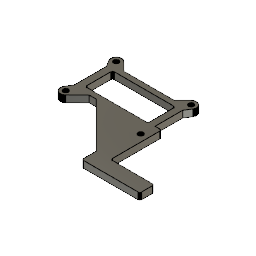
Plate (Autodesk Fusion 360 design; units mm, degrees)
Autodesk Fusion 360 part; units mm, degrees
(part 1 of 3)
sketch "Sketch1" plane through (0, 0, 0) normal (0, 0, 1) x (1, 0, 0)
  line L0 (57.3482, -23.9414) -> (57.363, -23.941)
  line L1 (57.363, -23.941) -> (57.3775, -23.9403)
  line L2 (57.3775, -23.9403) -> (57.3921, -23.9394)
  line L3 (57.3921, -23.9394) -> (57.4066, -23.9383)
  line L4 (57.4066, -23.9383) -> (57.4215, -23.9369)
  line L5 (57.4215, -23.9369) -> (57.436, -23.9352)
  line L6 (57.436, -23.9352) -> (57.4506, -23.9333)
  line L7 (57.4506, -23.9333) -> (57.4649, -23.9311)
  line L8 (57.4649, -23.9311) -> (57.4794, -23.9287)
  line L9 (57.4794, -23.9287) -> (57.494, -23.9261)
  line L10 (57.494, -23.9261) -> (57.5082, -23.9231)
  line L11 (57.5082, -23.9231) -> (57.5225, -23.9199)
  line L12 (57.5225, -23.9199) -> (57.5368, -23.9165)
  line L13 (57.5368, -23.9165) -> (57.5508, -23.9129)
  line L14 (57.5508, -23.9129) -> (57.5651, -23.9089)
  line L15 (57.5651, -23.9089) -> (57.5792, -23.9048)
  line L16 (57.5792, -23.9048) -> (57.5932, -23.9004)
  line L17 (57.5932, -23.9004) -> (57.6069, -23.8957)
  line L18 (57.6069, -23.8957) -> (57.621, -23.8908)
  line L19 (57.621, -23.8908) -> (57.6347, -23.8857)
  line L20 (57.6347, -23.8857) -> (57.6482, -23.8803)
  line L21 (57.6482, -23.8803) -> (57.6617, -23.8747)
  line L22 (57.6617, -23.8747) -> (57.6752, -23.8689)
  line L23 (57.6752, -23.8689) -> (57.6887, -23.8628)
  line L24 (57.6887, -23.8628) -> (57.7019, -23.8565)
  line L25 (57.7019, -23.8565) -> (57.7149, -23.8499)
  line L26 (57.7149, -23.8499) -> (57.7279, -23.8431)
  line L27 (57.7279, -23.8431) -> (57.7408, -23.8362)
  line L28 (57.7408, -23.8362) -> (57.7535, -23.8289)
  line L29 (57.7535, -23.8289) -> (57.7662, -23.8215)
  line L30 (57.7662, -23.8215) -> (57.7787, -23.8138)
  line L31 (57.7787, -23.8138) -> (57.7911, -23.806)
  line L32 (57.7911, -23.806) -> (57.8033, -23.7979)
  line L33 (57.8033, -23.7979) -> (57.8154, -23.7896)
  line L34 (57.8154, -23.7896) -> (57.8273, -23.781)
  line L35 (57.8273, -23.781) -> (57.839, -23.7723)
  line L36 (57.839, -23.7723) -> (57.8506, -23.7634)
  line L37 (57.8506, -23.7634) -> (57.8623, -23.7543)
  line L38 (57.8623, -23.7543) -> (57.8736, -23.745)
  line L39 (57.8736, -23.745) -> (57.8847, -23.7354)
  line L40 (57.8847, -23.7354) -> (57.8956, -23.7257)
  line L41 (57.8956, -23.7257) -> (57.9064, -23.7158)
  line L42 (57.9064, -23.7158) -> (57.917, -23.7057)
  line L43 (57.917, -23.7057) -> (57.9276, -23.6954)
  line L44 (57.9276, -23.6954) -> (57.9379, -23.685)
  line L45 (57.9379, -23.685) -> (57.948, -23.6743)
  line L46 (57.948, -23.6743) -> (57.9578, -23.6635)
  line L47 (57.9578, -23.6635) -> (57.9676, -23.6526)
  line L48 (57.9676, -23.6526) -> (57.9771, -23.6414)
  line L49 (57.9771, -23.6414) -> (57.9863, -23.6301)
  line L50 (57.9863, -23.6301) -> (57.9956, -23.6186)
  line L51 (57.9956, -23.6186) -> (58.0043, -23.607)
  line L52 (58.0043, -23.607) -> (58.0131, -23.5952)
  line L53 (58.0131, -23.5952) -> (58.0218, -23.5833)
  line L54 (58.0218, -23.5833) -> (58.03, -23.5712)
  line L55 (58.03, -23.5712) -> (58.0382, -23.559)
  line L56 (58.0382, -23.559) -> (58.0459, -23.5466)
  line L57 (58.0459, -23.5466) -> (58.0536, -23.5341)
  line L58 (58.0536, -23.5341) -> (58.061, -23.5215)
  line L59 (58.061, -23.5215) -> (58.0684, -23.5087)
  line L60 (58.0684, -23.5087) -> (58.0752, -23.4958)
  line L61 (58.0752, -23.4958) -> (58.0821, -23.4828)
  line L62 (58.0821, -23.4828) -> (58.0885, -23.4697)
  line L63 (58.0885, -23.4697) -> (58.0948, -23.4564)
  line L64 (58.0948, -23.4564) -> (58.1009, -23.4431)
  line L65 (58.1009, -23.4431) -> (58.1067, -23.4297)
  line L66 (58.1067, -23.4297) -> (58.1126, -23.4161)
  line L67 (58.1126, -23.4161) -> (58.1178, -23.4025)
  line L68 (58.1178, -23.4025) -> (58.1229, -23.3887)
  line L69 (58.1229, -23.3887) -> (58.1279, -23.3749)
  line L70 (58.1279, -23.3749) -> (58.1324, -23.361)
  line L71 (58.1324, -23.361) -> (58.1369, -23.347)
  line L72 (58.1369, -23.347) -> (58.1411, -23.333)
  line L73 (58.1411, -23.333) -> (58.1451, -23.3188)
  line L74 (58.1451, -23.3188) -> (58.1485, -23.3047)
  line L75 (58.1485, -23.3047) -> (58.152, -23.2904)
  line L76 (58.152, -23.2904) -> (58.1552, -23.2761)
  line L77 (58.1552, -23.2761) -> (58.1581, -23.2617)
  line L78 (58.1581, -23.2617) -> (58.1607, -23.2473)
  line L79 (58.1607, -23.2473) -> (58.1634, -23.2328)
  line L80 (58.1634, -23.2328) -> (58.1655, -23.2184)
  line L81 (58.1655, -23.2184) -> (58.1673, -23.2038)
  line L82 (58.1673, -23.2038) -> (58.1689, -23.1892)
  line L83 (58.1689, -23.1892) -> (58.1705, -23.1746)
  line L84 (58.1705, -23.1746) -> (58.1716, -23.16)
  line L85 (58.1716, -23.16) -> (58.1723, -23.1454)
  line L86 (58.1723, -23.1454) -> (58.1731, -23.1307)
  line L87 (58.1731, -23.1307) -> (58.1734, -23.1161)
  line L88 (58.1734, -23.1161) -> (58.1737, -23.1014)
  line L89 (58.1737, -23.1014) -> (58.1737, -18.0611)
  line L90 (58.1737, -18.0611) -> (58.1734, -18.0465)
  line L91 (58.1734, -18.0465) -> (58.1731, -18.0318)
  line L92 (58.1731, -18.0318) -> (58.1723, -18.0171)
  line L93 (58.1723, -18.0171) -> (58.1716, -18.0025)
  line L94 (58.1716, -18.0025) -> (58.1705, -17.9879)
  line L95 (58.1705, -17.9879) -> (58.1689, -17.9733)
  line L96 (58.1689, -17.9733) -> (58.1673, -17.9588)
  line L97 (58.1673, -17.9588) -> (58.1655, -17.9442)
  line L98 (58.1655, -17.9442) -> (58.1634, -17.9297)
  line L99 (58.1634, -17.9297) -> (58.1607, -17.9153)
  line L100 (58.1607, -17.9153) -> (58.1581, -17.9008)
  line L101 (58.1581, -17.9008) -> (58.1552, -17.8865)
  line L102 (58.1552, -17.8865) -> (58.152, -17.8722)
  line L103 (58.152, -17.8722) -> (58.1485, -17.8579)
  line L104 (58.1485, -17.8579) -> (58.1451, -17.8437)
  line L105 (58.1451, -17.8437) -> (58.1411, -17.8296)
  line L106 (58.1411, -17.8296) -> (58.1369, -17.8155)
  line L107 (58.1369, -17.8155) -> (58.1324, -17.8015)
  line L108 (58.1324, -17.8015) -> (58.1279, -17.7876)
  line L109 (58.1279, -17.7876) -> (58.1229, -17.7738)
  line L110 (58.1229, -17.7738) -> (58.1178, -17.7601)
  line L111 (58.1178, -17.7601) -> (58.1126, -17.7464)
  line L112 (58.1126, -17.7464) -> (58.1067, -17.7329)
  line L113 (58.1067, -17.7329) -> (58.1009, -17.7194)
  line L114 (58.1009, -17.7194) -> (58.0948, -17.7061)
  line L115 (58.0948, -17.7061) -> (58.0885, -17.6929)
  line L116 (58.0885, -17.6929) -> (58.0821, -17.6797)
  line L117 (58.0821, -17.6797) -> (58.0752, -17.6667)
  line L118 (58.0752, -17.6667) -> (58.0684, -17.6538)
  line L119 (58.0684, -17.6538) -> (58.061, -17.6411)
  line L120 (58.061, -17.6411) -> (58.0536, -17.6285)
  line L121 (58.0536, -17.6285) -> (58.0459, -17.616)
  line L122 (58.0459, -17.616) -> (58.0382, -17.6036)
  line L123 (58.0382, -17.6036) -> (58.03, -17.5914)
  line L124 (58.03, -17.5914) -> (58.0218, -17.5793)
  line L125 (58.0218, -17.5793) -> (58.0131, -17.5674)
  line L126 (58.0131, -17.5674) -> (58.0043, -17.5556)
  line L127 (58.0043, -17.5556) -> (57.9956, -17.5439)
  line L128 (57.9956, -17.5439) -> (57.9863, -17.5325)
  line L129 (57.9863, -17.5325) -> (57.9771, -17.5211)
  line L130 (57.9771, -17.5211) -> (57.9676, -17.51)
  line L131 (57.9676, -17.51) -> (57.9578, -17.499)
  line L132 (57.9578, -17.499) -> (57.948, -17.4882)
  line L133 (57.948, -17.4882) -> (57.9379, -17.4776)
  line L134 (57.9379, -17.4776) -> (57.9276, -17.4671)
  line L135 (57.9276, -17.4671) -> (57.917, -17.4568)
  line L136 (57.917, -17.4568) -> (57.9064, -17.4467)
  line L137 (57.9064, -17.4467) -> (57.8956, -17.4368)
  line L138 (57.8956, -17.4368) -> (57.8847, -17.4271)
  line L139 (57.8847, -17.4271) -> (57.8736, -17.4176)
  line L140 (57.8736, -17.4176) -> (57.8623, -17.4083)
  line L141 (57.8623, -17.4083) -> (57.8506, -17.3992)
  line L142 (57.8506, -17.3992) -> (57.839, -17.3902)
  line L143 (57.839, -17.3902) -> (57.8273, -17.3815)
  line L144 (57.8273, -17.3815) -> (57.8154, -17.373)
  line L145 (57.8154, -17.373) -> (57.8033, -17.3647)
  line L146 (57.8033, -17.3647) -> (57.7911, -17.3566)
  line L147 (57.7911, -17.3566) -> (57.7787, -17.3487)
  line L148 (57.7787, -17.3487) -> (57.7662, -17.3411)
  line L149 (57.7662, -17.3411) -> (57.7535, -17.3336)
  line L150 (57.7535, -17.3336) -> (57.7408, -17.3264)
  line L151 (57.7408, -17.3264) -> (57.7279, -17.3194)
  line L152 (57.7279, -17.3194) -> (57.7149, -17.3126)
  line L153 (57.7149, -17.3126) -> (57.7019, -17.3061)
  line L154 (57.7019, -17.3061) -> (57.6887, -17.2998)
  line L155 (57.6887, -17.2998) -> (57.6752, -17.2937)
  line L156 (57.6752, -17.2937) -> (57.6617, -17.2878)
  line L157 (57.6617, -17.2878) -> (57.6482, -17.2822)
  line L158 (57.6482, -17.2822) -> (57.6347, -17.2769)
  line L159 (57.6347, -17.2769) -> (57.621, -17.2717)
  line L160 (57.621, -17.2717) -> (57.6069, -17.2668)
  line L161 (57.6069, -17.2668) -> (57.5932, -17.2622)
  line L162 (57.5932, -17.2622) -> (57.5792, -17.2578)
  line L163 (57.5792, -17.2578) -> (57.5651, -17.2536)
  line L164 (57.5651, -17.2536) -> (57.5508, -17.2497)
  line L165 (57.5508, -17.2497) -> (57.5368, -17.246)
  line L166 (57.5368, -17.246) -> (57.5225, -17.2426)
  line L167 (57.5225, -17.2426) -> (57.5082, -17.2394)
  line L168 (57.5082, -17.2394) -> (57.494, -17.2365)
  line L169 (57.494, -17.2365) -> (57.4794, -17.2338)
  line L170 (57.4794, -17.2338) -> (57.4649, -17.2314)
  line L171 (57.4649, -17.2314) -> (57.4506, -17.2292)
  line L172 (57.4506, -17.2292) -> (57.436, -17.2273)
  line L173 (57.436, -17.2273) -> (57.4215, -17.2257)
  line L174 (57.4215, -17.2257) -> (57.4066, -17.2243)
  line L175 (57.4066, -17.2243) -> (57.3921, -17.2231)
  line L176 (57.3921, -17.2231) -> (57.3775, -17.2222)
  line L177 (57.3775, -17.2222) -> (57.363, -17.2216)
  line L178 (57.363, -17.2216) -> (57.3482, -17.2212)
  line L179 (57.3482, -17.2212) -> (57.3336, -17.2211)
  line L180 (57.3336, -17.2211) -> (38.8562, -17.2211)
  line L181 (38.8562, -17.2211) -> (38.8379, -17.2209)
  line L182 (38.8379, -17.2209) -> (38.8231, -17.2205)
  line L183 (38.8231, -17.2205) -> (38.8083, -17.2199)
  line L184 (38.8083, -17.2199) -> (38.7937, -17.219)
  line L185 (38.7937, -17.219) -> (38.7792, -17.2178)
  line L186 (38.7792, -17.2178) -> (38.7646, -17.2164)
  line L187 (38.7646, -17.2164) -> (38.7501, -17.2148)
  line L188 (38.7501, -17.2148) -> (38.7355, -17.2129)
  line L189 (38.7355, -17.2129) -> (38.721, -17.2107)
  line L190 (38.721, -17.2107) -> (38.7064, -17.2082)
  line L191 (38.7064, -17.2082) -> (38.6921, -17.2056)
  line L192 (38.6921, -17.2056) -> (38.6779, -17.2027)
  line L193 (38.6779, -17.2027) -> (38.6636, -17.1995)
  line L194 (38.6636, -17.1995) -> (38.649, -17.196)
  line L195 (38.649, -17.196) -> (38.635, -17.1924)
  line L196 (38.635, -17.1924) -> (38.621, -17.1885)
  line L197 (38.621, -17.1885) -> (38.6067, -17.1843)
  line L198 (38.6067, -17.1843) -> (38.5929, -17.18)
  line L199 (38.5929, -17.18) -> (38.5789, -17.1753)
  line L200 (38.5789, -17.1753) -> (38.5651, -17.1704)
  line L201 (38.5651, -17.1704) -> (38.5514, -17.1652)
  line L202 (38.5514, -17.1652) -> (38.5379, -17.1599)
  line L203 (38.5379, -17.1599) -> (38.5241, -17.1542)
  line L204 (38.5241, -17.1542) -> (38.5109, -17.1484)
  line L205 (38.5109, -17.1484) -> (38.4974, -17.1423)
  line L206 (38.4974, -17.1423) -> (38.4842, -17.136)
  line L207 (38.4842, -17.136) -> (38.4709, -17.1294)
  line L208 (38.4709, -17.1294) -> (38.4582, -17.1228)
  line L209 (38.4582, -17.1228) -> (38.445, -17.1157)
  line L210 (38.445, -17.1157) -> (38.4326, -17.1085)
  line L211 (38.4326, -17.1085) -> (38.4199, -17.1011)
  line L212 (38.4199, -17.1011) -> (38.4072, -17.0934)
  line L213 (38.4072, -17.0934) -> (38.395, -17.0855)
  line L214 (38.395, -17.0855) -> (38.3826, -17.0774)
  line L215 (38.3826, -17.0774) -> (38.3707, -17.0692)
  line L216 (38.3707, -17.0692) -> (38.3585, -17.0606)
  line L217 (38.3585, -17.0606) -> (38.3469, -17.0519)
  line L218 (38.3469, -17.0519) -> (38.3352, -17.0429)
  line L219 (38.3352, -17.0429) -> (38.3238, -17.0338)
  line L220 (38.3238, -17.0338) -> (38.3125, -17.0246)
  line L221 (38.3125, -17.0246) -> (38.3013, -17.0149)
  line L222 (38.3013, -17.0149) -> (38.2902, -17.0053)
  line L223 (38.2902, -17.0053) -> (38.2794, -16.9953)
  line L224 (38.2794, -16.9953) -> (38.2688, -16.9853)
  line L225 (38.2688, -16.9853) -> (38.2585, -16.975)
  line L226 (38.2585, -16.975) -> (38.2482, -16.9645)
  line L227 (38.2482, -16.9645) -> (38.2381, -16.954)
  line L228 (38.2381, -16.954) -> (38.2281, -16.943)
  line L229 (38.2281, -16.943) -> (38.2185, -16.9322)
  line L230 (38.2185, -16.9322) -> (38.2087, -16.9208)
  line L231 (38.2087, -16.9208) -> (38.1995, -16.9097)
  line L232 (38.1995, -16.9097) -> (38.1905, -16.8982)
  line L233 (38.1905, -16.8982) -> (38.1815, -16.8865)
  line L234 (38.1815, -16.8865) -> (38.1728, -16.8748)
  line L235 (38.1728, -16.8748) -> (38.1643, -16.8628)
  line L236 (38.1643, -16.8628) -> (38.1561, -16.8508)
  line L237 (38.1561, -16.8508) -> (38.1479, -16.8385)
  line L238 (38.1479, -16.8385) -> (38.14, -16.8262)
  line L239 (38.14, -16.8262) -> (38.1323, -16.8137)
  line L240 (38.1323, -16.8137) -> (38.1249, -16.801)
  line L241 (38.1249, -16.801) -> (38.1177, -16.7884)
  line L242 (38.1177, -16.7884) -> (38.1106, -16.7752)
  line L243 (38.1106, -16.7752) -> (38.104, -16.7625)
  line L244 (38.104, -16.7625) -> (38.0974, -16.7493)
  line L245 (38.0974, -16.7493) -> (38.091, -16.7361)
  line L246 (38.091, -16.7361) -> (38.0849, -16.7226)
  line L247 (38.0849, -16.7226) -> (38.0791, -16.7093)
  line L248 (38.0791, -16.7093) -> (38.0735, -16.6956)
  line L249 (38.0735, -16.6956) -> (38.0683, -16.6821)
  line L250 (38.0683, -16.6821) -> (38.063, -16.6683)
  line L251 (38.063, -16.6683) -> (38.0582, -16.6545)
  line L252 (38.0582, -16.6545) -> (38.0534, -16.6405)
  line L253 (38.0534, -16.6405) -> (38.0492, -16.6266)
  line L254 (38.0492, -16.6266) -> (38.045, -16.6125)
  line L255 (38.045, -16.6125) -> (38.041, -16.5984)
  line L256 (38.041, -16.5984) -> (38.0373, -16.5844)
  line L257 (38.0373, -16.5844) -> (38.0339, -16.5699)
  line L258 (38.0339, -16.5699) -> (38.0307, -16.5555)
  line L259 (38.0307, -16.5555) -> (38.0278, -16.5414)
  line L260 (38.0278, -16.5414) -> (38.0251, -16.527)
  line L261 (38.0251, -16.527) -> (38.0227, -16.5123)
  line L262 (38.0227, -16.5123) -> (38.0206, -16.4979)
  line L263 (38.0206, -16.4979) -> (38.0188, -16.4834)
  line L264 (38.0188, -16.4834) -> (38.0169, -16.4687)
  line L265 (38.0169, -16.4687) -> (38.0156, -16.4543)
  line L266 (38.0156, -16.4543) -> (38.0145, -16.4396)
  line L267 (38.0145, -16.4396) -> (38.0135, -16.4252)
  line L268 (38.0135, -16.4252) -> (38.013, -16.4103)
  line L269 (38.013, -16.4103) -> (38.0124, -16.3956)
  line L270 (38.0124, -16.3956) -> (38.0124, -16.3773)
  line L271 (38.0124, -16.3773) -> (38.0124, 5.4603)
  line L272 (38.0124, 5.4603) -> (38.0122, 5.475)
  line L273 (38.0122, 5.475) -> (38.0119, 5.4897)
  line L274 (38.0119, 5.4897) -> (38.0111, 5.5043)
  line L275 (38.0111, 5.5043) -> (38.0103, 5.5189)
  line L276 (38.0103, 5.5189) -> (38.0092, 5.5335)
  line L277 (38.0092, 5.5335) -> (38.0077, 5.5482)
  line L278 (38.0077, 5.5482) -> (38.0061, 5.5627)
  line L279 (38.0061, 5.5627) -> (38.0042, 5.5773)
  line L280 (38.0042, 5.5773) -> (38.0021, 5.5918)
  line L281 (38.0021, 5.5918) -> (37.9995, 5.6062)
  line L282 (37.9995, 5.6062) -> (37.9968, 5.6206)
  line L283 (37.9968, 5.6206) -> (37.9939, 5.635)
  line L284 (37.9939, 5.635) -> (37.9907, 5.6493)
  line L285 (37.9907, 5.6493) -> (37.9873, 5.6636)
  line L286 (37.9873, 5.6636) -> (37.9838, 5.6777)
  line L287 (37.9838, 5.6777) -> (37.9799, 5.6919)
  line L288 (37.9799, 5.6919) -> (37.9756, 5.706)
  line L289 (37.9756, 5.706) -> (37.9711, 5.7199)
  line L290 (37.9711, 5.7199) -> (37.9667, 5.7338)
  line L291 (37.9667, 5.7338) -> (37.9616, 5.7476)
  line L292 (37.9616, 5.7476) -> (37.9566, 5.7614)
  line L293 (37.9566, 5.7614) -> (37.9513, 5.775)
  line L294 (37.9513, 5.775) -> (37.9455, 5.7886)
  line L295 (37.9455, 5.7886) -> (37.9397, 5.802)
  line L296 (37.9397, 5.802) -> (37.9336, 5.8154)
  line L297 (37.9336, 5.8154) -> (37.9272, 5.8286)
  line L298 (37.9272, 5.8286) -> (37.9209, 5.8417)
  line L299 (37.9209, 5.8417) -> (37.914, 5.8547)
  line L300 (37.914, 5.8547) -> (37.9071, 5.8676)
  line L301 (37.9071, 5.8676) -> (37.8997, 5.8804)
  line L302 (37.8997, 5.8804) -> (37.8923, 5.893)
  line L303 (37.8923, 5.893) -> (37.8846, 5.9055)
  line L304 (37.8846, 5.9055) -> (37.877, 5.9179)
  line L305 (37.877, 5.9179) -> (37.8688, 5.9301)
  line L306 (37.8688, 5.9301) -> (37.8606, 5.9422)
  line L307 (37.8606, 5.9422) -> (37.8518, 5.9541)
  line L308 (37.8518, 5.9541) -> (37.8431, 5.9659)
  line L309 (37.8431, 5.9659) -> (37.8344, 5.9775)
  line L310 (37.8344, 5.9775) -> (37.8251, 5.989)
  line L311 (37.8251, 5.989) -> (37.8158, 6.0003)
  line L312 (37.8158, 6.0003) -> (37.8063, 6.0115)
  line L313 (37.8063, 6.0115) -> (37.7965, 6.0224)
  line L314 (37.7965, 6.0224) -> (37.7867, 6.0332)
  line L315 (37.7867, 6.0332) -> (37.7767, 6.0439)
  line L316 (37.7767, 6.0439) -> (37.7664, 6.0544)
  line L317 (37.7664, 6.0544) -> (37.7558, 6.0646)
  line L318 (37.7558, 6.0646) -> (37.7452, 6.0747)
  line L319 (37.7452, 6.0747) -> (37.7343, 6.0846)
  line L320 (37.7343, 6.0846) -> (37.7235, 6.0943)
  line L321 (37.7235, 6.0943) -> (37.7124, 6.1039)
  line L322 (37.7124, 6.1039) -> (37.701, 6.1132)
  line L323 (37.701, 6.1132) -> (37.6894, 6.1223)
  line L324 (37.6894, 6.1223) -> (37.6777, 6.1312)
  line L325 (37.6777, 6.1312) -> (37.6661, 6.1399)
  line L326 (37.6661, 6.1399) -> (37.6542, 6.1485)
  line L327 (37.6542, 6.1485) -> (37.642, 6.1568)
  line L328 (37.642, 6.1568) -> (37.6298, 6.1649)
  line L329 (37.6298, 6.1649) -> (37.6174, 6.1727)
  line L330 (37.6174, 6.1727) -> (37.605, 6.1804)
  line L331 (37.605, 6.1804) -> (37.5923, 6.1878)
  line L332 (37.5923, 6.1878) -> (37.5796, 6.1951)
  line L333 (37.5796, 6.1951) -> (37.5666, 6.202)
  line L334 (37.5666, 6.202) -> (37.5536, 6.2088)
  line L335 (37.5536, 6.2088) -> (37.5407, 6.2154)
  line L336 (37.5407, 6.2154) -> (37.5274, 6.2217)
  line L337 (37.5274, 6.2217) -> (37.5139, 6.2278)
  line L338 (37.5139, 6.2278) -> (37.5005, 6.2336)
  line L339 (37.5005, 6.2336) -> (37.487, 6.2392)
  line L340 (37.487, 6.2392) -> (37.4735, 6.2446)
  line L341 (37.4735, 6.2446) -> (37.4597, 6.2497)
  line L342 (37.4597, 6.2497) -> (37.4457, 6.2546)
  line L343 (37.4457, 6.2546) -> (37.4319, 6.2593)
  line L344 (37.4319, 6.2593) -> (37.4179, 6.2637)
  line L345 (37.4179, 6.2637) -> (37.4039, 6.2678)
  line L346 (37.4039, 6.2678) -> (37.3896, 6.2718)
  line L347 (37.3896, 6.2718) -> (37.3756, 6.2754)
  line L348 (37.3756, 6.2754) -> (37.3613, 6.2789)
  line L349 (37.3613, 6.2789) -> (37.347, 6.282)
  line L350 (37.347, 6.282) -> (37.3327, 6.285)
  line L351 (37.3327, 6.285) -> (37.3182, 6.2876)
  line L352 (37.3182, 6.2876) -> (37.3036, 6.29)
  line L353 (37.3036, 6.29) -> (37.2893, 6.2922)
  line L354 (37.2893, 6.2922) -> (37.2748, 6.2941)
  line L355 (37.2748, 6.2941) -> (37.2602, 6.2958)
  line L356 (37.2602, 6.2958) -> (37.2454, 6.2972)
  line L357 (37.2454, 6.2972) -> (37.2308, 6.2983)
  line L358 (37.2308, 6.2983) -> (37.2163, 6.2992)
  line L359 (37.2163, 6.2992) -> (37.2017, 6.2999)
  line L360 (37.2017, 6.2999) -> (37.1869, 6.3003)
  line L361 (37.1869, 6.3003) -> (37.1724, 6.3004)
  line L362 (37.1724, 6.3004) -> (34.9671, 6.3004)
  line L363 (34.9671, 6.3004) -> (34.9671, 19.1018)
  line L364 (34.9671, 19.1018) -> (36.7893, 21.976)
  line L365 (36.7893, 21.976) -> (36.8123, 22.0135)
  line L366 (36.8123, 22.0135) -> (36.8348, 22.0514)
  line L367 (36.8348, 22.0514) -> (36.8562, 22.0896)
  line L368 (36.8562, 22.0896) -> (36.8774, 22.1283)
  line L369 (36.8774, 22.1283) -> (36.8977, 22.1673)
  line L370 (36.8977, 22.1673) -> (36.9173, 22.2067)
  line L371 (36.9173, 22.2067) -> (36.9361, 22.2464)
  line L372 (36.9361, 22.2464) -> (36.9544, 22.2864)
  line L373 (36.9544, 22.2864) -> (36.9721, 22.3267)
  line L374 (36.9721, 22.3267) -> (36.9888, 22.3674)
  line L375 (36.9888, 22.3674) -> (37.0049, 22.4083)
  line L376 (37.0049, 22.4083) -> (37.0202, 22.4495)
  line L377 (37.0202, 22.4495) -> (37.0351, 22.491)
  line L378 (37.0351, 22.491) -> (37.0491, 22.5327)
  line L379 (37.0491, 22.5327) -> (37.0623, 22.5746)
  line L380 (37.0623, 22.5746) -> (37.0747, 22.6168)
  line L381 (37.0747, 22.6168) -> (37.0864, 22.6592)
  line L382 (37.0864, 22.6592) -> (37.0975, 22.7018)
  line L383 (37.0975, 22.7018) -> (37.1078, 22.7445)
  line L384 (37.1078, 22.7445) -> (37.1173, 22.7875)
  line L385 (37.1173, 22.7875) -> (37.1261, 22.8306)
  line L386 (37.1261, 22.8306) -> (37.134, 22.8738)
  line L387 (37.134, 22.8738) -> (37.1412, 22.9172)
  line L388 (37.1412, 22.9172) -> (37.1478, 22.9607)
  line L389 (37.1478, 22.9607) -> (37.1536, 23.0043)
  line L390 (37.1536, 23.0043) -> (37.1586, 23.048)
  line L391 (37.1586, 23.048) -> (37.1628, 23.0918)
  line L392 (37.1628, 23.0918) -> (37.1663, 23.1356)
  line L393 (37.1663, 23.1356) -> (37.1689, 23.1795)
  line L394 (37.1689, 23.1795) -> (37.1708, 23.2235)
  line L395 (37.1708, 23.2235) -> (37.1718, 23.2675)
  line L396 (37.1718, 23.2675) -> (37.1724, 23.3114)
  line L397 (37.1724, 23.3114) -> (37.1718, 23.3554)
  line L398 (37.1718, 23.3554) -> (37.1708, 23.3994)
  line L399 (37.1708, 23.3994) -> (37.1689, 23.4433)
  line L400 (37.1689, 23.4433) -> (37.1663, 23.4872)
  line L401 (37.1663, 23.4872) -> (37.1628, 23.5311)
  line L402 (37.1628, 23.5311) -> (37.1586, 23.5749)
  line L403 (37.1586, 23.5749) -> (37.1536, 23.6186)
  line L404 (37.1536, 23.6186) -> (37.1478, 23.6622)
  line L405 (37.1478, 23.6622) -> (37.1412, 23.7057)
  line L406 (37.1412, 23.7057) -> (37.134, 23.7491)
  line L407 (37.134, 23.7491) -> (37.1261, 23.7923)
  line L408 (37.1261, 23.7923) -> (37.1173, 23.8354)
  line L409 (37.1173, 23.8354) -> (37.1078, 23.8784)
  line L410 (37.1078, 23.8784) -> (37.0975, 23.9211)
  line L411 (37.0975, 23.9211) -> (37.0864, 23.9637)
  line L412 (37.0864, 23.9637) -> (37.0747, 24.0061)
  line L413 (37.0747, 24.0061) -> (37.0623, 24.0483)
  line L414 (37.0623, 24.0483) -> (37.0491, 24.0902)
  line L415 (37.0491, 24.0902) -> (37.0351, 24.1319)
  line L416 (37.0351, 24.1319) -> (37.0202, 24.1734)
  line L417 (37.0202, 24.1734) -> (37.0049, 24.2146)
  line L418 (37.0049, 24.2146) -> (36.9888, 24.2555)
  line L419 (36.9888, 24.2555) -> (36.9721, 24.2962)
  line L420 (36.9721, 24.2962) -> (36.9544, 24.3365)
  line L421 (36.9544, 24.3365) -> (36.9361, 24.3765)
  line L422 (36.9361, 24.3765) -> (36.9173, 24.4162)
  line L423 (36.9173, 24.4162) -> (36.8977, 24.4556)
  line L424 (36.8977, 24.4556) -> (36.8774, 24.4946)
  line L425 (36.8774, 24.4946) -> (36.8562, 24.5333)
  line L426 (36.8562, 24.5333) -> (36.8348, 24.5715)
  line L427 (36.8348, 24.5715) -> (36.8123, 24.6094)
  line L428 (36.8123, 24.6094) -> (36.7893, 24.6469)
  line L429 (36.7893, 24.6469) -> (36.7657, 24.684)
  line L430 (36.7657, 24.684) -> (36.7414, 24.7207)
  line L431 (36.7414, 24.7207) -> (36.7165, 24.757)
  line L432 (36.7165, 24.757) -> (36.6911, 24.7928)
  line L433 (36.6911, 24.7928) -> (36.6649, 24.8281)
  line L434 (36.6649, 24.8281) -> (36.6382, 24.863)
  line L435 (36.6382, 24.863) -> (36.6107, 24.8974)
  line L436 (36.6107, 24.8974) -> (36.5826, 24.9314)
  line L437 (36.5826, 24.9314) -> (36.554, 24.9648)
  line L438 (36.554, 24.9648) -> (36.5249, 24.9978)
  line L439 (36.5249, 24.9978) -> (36.4953, 25.0302)
  line L440 (36.4953, 25.0302) -> (36.4649, 25.0621)
  line L441 (36.4649, 25.0621) -> (36.4342, 25.0935)
  line L442 (36.4342, 25.0935) -> (36.4027, 25.1243)
  line L443 (36.4027, 25.1243) -> (36.3709, 25.1546)
  line L444 (36.3709, 25.1546) -> (36.3384, 25.1843)
  line L445 (36.3384, 25.1843) -> (36.3056, 25.2134)
  line L446 (36.3056, 25.2134) -> (36.272, 25.242)
  line L447 (36.272, 25.242) -> (36.2381, 25.27)
  line L448 (36.2381, 25.27) -> (36.2037, 25.2973)
  line L449 (36.2037, 25.2973) -> (36.1688, 25.3241)
  line L450 (36.1688, 25.3241) -> (36.1334, 25.3503)
  line L451 (36.1334, 25.3503) -> (36.0976, 25.3758)
  line L452 (36.0976, 25.3758) -> (36.0614, 25.4007)
  line L453 (36.0614, 25.4007) -> (36.0246, 25.425)
  line L454 (36.0246, 25.425) -> (35.9876, 25.4487)
  line L455 (35.9876, 25.4487) -> (35.95, 25.4716)
  line L456 (35.95, 25.4716) -> (35.9122, 25.494)
  line L457 (35.9122, 25.494) -> (35.8741, 25.5156)
  line L458 (35.8741, 25.5156) -> (35.8352, 25.5366)
  line L459 (35.8352, 25.5366) -> (35.7963, 25.5569)
  line L460 (35.7963, 25.5569) -> (35.7568, 25.5766)
  line L461 (35.7568, 25.5766) -> (35.7172, 25.5955)
  line L462 (35.7172, 25.5955) -> (35.6772, 25.6137)
  line L463 (35.6772, 25.6137) -> (35.6367, 25.6313)
  line L464 (35.6367, 25.6313) -> (35.5962, 25.6481)
  line L465 (35.5962, 25.6481) -> (35.5552, 25.6642)
  line L466 (35.5552, 25.6642) -> (35.514, 25.6796)
  line L467 (35.514, 25.6796) -> (35.4727, 25.6943)
  line L468 (35.4727, 25.6943) -> (35.4309, 25.7083)
  line L469 (35.4309, 25.7083) -> (35.3891, 25.7215)
  line L470 (35.3891, 25.7215) -> (35.3467, 25.734)
  line L471 (35.3467, 25.734) -> (35.3044, 25.7457)
  line L472 (35.3044, 25.7457) -> (35.2618, 25.7567)
  line L473 (35.2618, 25.7567) -> (35.219, 25.767)
  line L474 (35.219, 25.767) -> (35.1761, 25.7765)
  line L475 (35.1761, 25.7765) -> (35.133, 25.7853)
  line L476 (35.133, 25.7853) -> (35.0898, 25.7933)
  line L477 (35.0898, 25.7933) -> (35.0464, 25.8006)
  line L478 (35.0464, 25.8006) -> (35.0028, 25.8071)
  line L479 (35.0028, 25.8071) -> (34.9594, 25.8128)
  line L480 (34.9594, 25.8128) -> (34.9155, 25.8178)
  line L481 (34.9155, 25.8178) -> (34.8718, 25.822)
  line L482 (34.8718, 25.822) -> (34.8279, 25.8255)
  line L483 (34.8279, 25.8255) -> (34.784, 25.8281)
  line L484 (34.784, 25.8281) -> (34.7401, 25.8301)
  line L485 (34.7401, 25.8301) -> (34.6961, 25.8312)
  line L486 (34.6961, 25.8312) -> (34.6522, 25.8316)
  line L487 (34.6522, 25.8316) -> (34.6083, 25.8312)
  line L488 (34.6083, 25.8312) -> (34.5641, 25.8301)
  line L489 (34.5641, 25.8301) -> (34.5202, 25.8281)
  line L490 (34.5202, 25.8281) -> (34.4763, 25.8255)
  line L491 (34.4763, 25.8255) -> (34.4326, 25.822)
  line L492 (34.4326, 25.822) -> (34.3887, 25.8178)
  line L493 (34.3887, 25.8178) -> (34.345, 25.8128)
  line L494 (34.345, 25.8128) -> (34.3014, 25.8071)
  line L495 (34.3014, 25.8071) -> (34.258, 25.8006)
  line L496 (34.258, 25.8006) -> (34.2146, 25.7933)
  line L497 (34.2146, 25.7933) -> (34.1712, 25.7853)
  line L498 (34.1712, 25.7853) -> (34.1281, 25.7765)
  line L499 (34.1281, 25.7765) -> (34.0852, 25.767)
  line L500 (34.0852, 25.767) -> (34.0424, 25.7567)
  line L501 (34.0424, 25.7567) -> (33.9998, 25.7457)
  line L502 (33.9998, 25.7457) -> (33.9574, 25.734)
  line L503 (33.9574, 25.734) -> (33.9154, 25.7215)
  line L504 (33.9154, 25.7215) -> (33.8733, 25.7083)
  line L505 (33.8733, 25.7083) -> (33.8317, 25.6943)
  line L506 (33.8317, 25.6943) -> (33.7902, 25.6796)
  line L507 (33.7902, 25.6796) -> (33.7489, 25.6642)
  line L508 (33.7489, 25.6642) -> (33.7082, 25.6481)
  line L509 (33.7082, 25.6481) -> (33.6674, 25.6313)
  line L510 (33.6674, 25.6313) -> (33.6272, 25.6137)
  line L511 (33.6272, 25.6137) -> (33.587, 25.5955)
  line L512 (33.587, 25.5955) -> (33.5473, 25.5766)
  line L513 (33.5473, 25.5766) -> (33.5079, 25.5569)
  line L514 (33.5079, 25.5569) -> (33.469, 25.5366)
  line L515 (33.469, 25.5366) -> (33.4304, 25.5156)
  line L516 (33.4304, 25.5156) -> (33.392, 25.494)
  line L517 (33.392, 25.494) -> (33.3542, 25.4716)
  line L518 (33.3542, 25.4716) -> (33.3166, 25.4487)
  line L519 (33.3166, 25.4487) -> (33.2796, 25.425)
  line L520 (33.2796, 25.425) -> (33.2428, 25.4007)
  line L521 (33.2428, 25.4007) -> (33.2065, 25.3758)
  line L522 (33.2065, 25.3758) -> (33.1708, 25.3503)
  line L523 (33.1708, 25.3503) -> (33.1354, 25.3241)
  line L524 (33.1354, 25.3241) -> (33.1007, 25.2973)
  line L525 (33.1007, 25.2973) -> (33.066, 25.27)
  line L526 (33.066, 25.27) -> (33.0322, 25.242)
  line L527 (33.0322, 25.242) -> (32.9988, 25.2134)
  line L528 (32.9988, 25.2134) -> (32.9658, 25.1843)
  line L529 (32.9658, 25.1843) -> (32.9335, 25.1546)
  line L530 (32.9335, 25.1546) -> (32.9015, 25.1243)
  line L531 (32.9015, 25.1243) -> (28.902, 21.2113)
  line L532 (28.902, 21.2113) -> (5.75, 21.2113)
  line L533 (5.75, 21.2113) -> (1.7506, 25.1243)
  line L534 (1.7506, 25.1243) -> (1.7187, 25.1546)
  line L535 (1.7187, 25.1546) -> (1.6863, 25.1843)
  line L536 (1.6863, 25.1843) -> (1.6534, 25.2134)
  line L537 (1.6534, 25.2134) -> (1.6199, 25.242)
  line L538 (1.6199, 25.242) -> (1.586, 25.27)
  line L539 (1.586, 25.27) -> (1.5516, 25.2973)
  line L540 (1.5516, 25.2973) -> (1.5167, 25.3241)
  line L541 (1.5167, 25.3241) -> (1.4813, 25.3503)
  line L542 (1.4813, 25.3503) -> (1.4455, 25.3758)
  line L543 (1.4455, 25.3758) -> (1.4093, 25.4007)
  line L544 (1.4093, 25.4007) -> (1.3726, 25.425)
  line L545 (1.3726, 25.425) -> (1.3355, 25.4487)
  line L546 (1.3355, 25.4487) -> (1.298, 25.4716)
  line L547 (1.298, 25.4716) -> (1.2601, 25.494)
  line L548 (1.2601, 25.494) -> (1.2218, 25.5156)
  line L549 (1.2218, 25.5156) -> (1.1831, 25.5366)
  line L550 (1.1831, 25.5366) -> (1.1441, 25.5569)
  line L551 (1.1441, 25.5569) -> (1.1048, 25.5766)
  line L552 (1.1048, 25.5766) -> (1.0651, 25.5955)
  line L553 (1.0651, 25.5955) -> (1.025, 25.6137)
  line L554 (1.025, 25.6137) -> (0.9847, 25.6313)
  line L555 (0.9847, 25.6313) -> (0.9441, 25.6481)
  line L556 (0.9441, 25.6481) -> (0.9031, 25.6642)
  line L557 (0.9031, 25.6642) -> (0.8619, 25.6796)
  line L558 (0.8619, 25.6796) -> (0.8205, 25.6943)
  line L559 (0.8205, 25.6943) -> (0.7788, 25.7083)
  line L560 (0.7788, 25.7083) -> (0.7368, 25.7215)
  line L561 (0.7368, 25.7215) -> (0.6946, 25.734)
  line L562 (0.6946, 25.734) -> (0.6523, 25.7457)
  line L563 (0.6523, 25.7457) -> (0.6097, 25.7567)
  line L564 (0.6097, 25.7567) -> (0.5669, 25.767)
  line L565 (0.5669, 25.767) -> (0.524, 25.7765)
  line L566 (0.524, 25.7765) -> (0.4809, 25.7853)
  line L567 (0.4809, 25.7853) -> (0.4376, 25.7933)
  line L568 (0.4376, 25.7933) -> (0.3942, 25.8006)
  line L569 (0.3942, 25.8006) -> (0.3507, 25.8071)
  line L570 (0.3507, 25.8071) -> (0.3071, 25.8128)
  line L571 (0.3071, 25.8128) -> (0.2634, 25.8178)
  line L572 (0.2634, 25.8178) -> (0.2196, 25.822)
  line L573 (0.2196, 25.822) -> (0.1758, 25.8255)
  line L574 (0.1758, 25.8255) -> (0.1319, 25.8281)
  line L575 (0.1319, 25.8281) -> (0.088, 25.8301)
  line L576 (0.088, 25.8301) -> (0.044, 25.8312)
  line L577 (0.044, 25.8312) -> (0, 25.8316)
  line L578 (0, 25.8316) -> (-0.044, 25.8312)
  line L579 (-0.044, 25.8312) -> (-0.088, 25.8301)
  line L580 (-0.088, 25.8301) -> (-0.1319, 25.8281)
  line L581 (-0.1319, 25.8281) -> (-0.1758, 25.8255)
  line L582 (-0.1758, 25.8255) -> (-0.2196, 25.822)
  line L583 (-0.2196, 25.822) -> (-0.2634, 25.8178)
  line L584 (-0.2634, 25.8178) -> (-0.3071, 25.8128)
  line L585 (-0.3071, 25.8128) -> (-0.3507, 25.8071)
  line L586 (-0.3507, 25.8071) -> (-0.3942, 25.8006)
  line L587 (-0.3942, 25.8006) -> (-0.4376, 25.7933)
  line L588 (-0.4376, 25.7933) -> (-0.4809, 25.7853)
  line L589 (-0.4809, 25.7853) -> (-0.524, 25.7765)
  line L590 (-0.524, 25.7765) -> (-0.5669, 25.767)
  line L591 (-0.5669, 25.767) -> (-0.6097, 25.7567)
  line L592 (-0.6097, 25.7567) -> (-0.6523, 25.7457)
  line L593 (-0.6523, 25.7457) -> (-0.6946, 25.734)
  line L594 (-0.6946, 25.734) -> (-0.7368, 25.7215)
  line L595 (-0.7368, 25.7215) -> (-0.7788, 25.7083)
  line L596 (-0.7788, 25.7083) -> (-0.8205, 25.6943)
  line L597 (-0.8205, 25.6943) -> (-0.8619, 25.6796)
  line L598 (-0.8619, 25.6796) -> (-0.9031, 25.6642)
  line L599 (-0.9031, 25.6642) -> (-0.9441, 25.6481)
  line L600 (-0.9441, 25.6481) -> (-0.9847, 25.6313)
  line L601 (-0.9847, 25.6313) -> (-1.025, 25.6137)
  line L602 (-1.025, 25.6137) -> (-1.0651, 25.5955)
  line L603 (-1.0651, 25.5955) -> (-1.1048, 25.5766)
  line L604 (-1.1048, 25.5766) -> (-1.1441, 25.5569)
  line L605 (-1.1441, 25.5569) -> (-1.1831, 25.5366)
  line L606 (-1.1831, 25.5366) -> (-1.2218, 25.5156)
  line L607 (-1.2218, 25.5156) -> (-1.2601, 25.494)
  line L608 (-1.2601, 25.494) -> (-1.298, 25.4716)
  line L609 (-1.298, 25.4716) -> (-1.3355, 25.4487)
  line L610 (-1.3355, 25.4487) -> (-1.3726, 25.425)
  line L611 (-1.3726, 25.425) -> (-1.4093, 25.4007)
  line L612 (-1.4093, 25.4007) -> (-1.4455, 25.3758)
  line L613 (-1.4455, 25.3758) -> (-1.4813, 25.3503)
  line L614 (-1.4813, 25.3503) -> (-1.5167, 25.3241)
  line L615 (-1.5167, 25.3241) -> (-1.5516, 25.2973)
  line L616 (-1.5516, 25.2973) -> (-1.586, 25.27)
  line L617 (-1.586, 25.27) -> (-1.6199, 25.242)
  line L618 (-1.6199, 25.242) -> (-1.6534, 25.2134)
  line L619 (-1.6534, 25.2134) -> (-1.6863, 25.1843)
  line L620 (-1.6863, 25.1843) -> (-1.7187, 25.1546)
  line L621 (-1.7187, 25.1546) -> (-1.7506, 25.1243)
  line L622 (-1.7506, 25.1243) -> (-1.782, 25.0935)
  line L623 (-1.782, 25.0935) -> (-1.8128, 25.0621)
  line L624 (-1.8128, 25.0621) -> (-1.8431, 25.0302)
  line L625 (-1.8431, 25.0302) -> (-1.8728, 24.9978)
  line L626 (-1.8728, 24.9978) -> (-1.902, 24.9648)
  line L627 (-1.902, 24.9648) -> (-1.9306, 24.9314)
  line L628 (-1.9306, 24.9314) -> (-1.9585, 24.8974)
  line L629 (-1.9585, 24.8974) -> (-1.9859, 24.863)
  line L630 (-1.9859, 24.863) -> (-2.0127, 24.8281)
  line L631 (-2.0127, 24.8281) -> (-2.0389, 24.7928)
  line L632 (-2.0389, 24.7928) -> (-2.0644, 24.757)
  line L633 (-2.0644, 24.757) -> (-2.0893, 24.7207)
  line L634 (-2.0893, 24.7207) -> (-2.1136, 24.684)
  line L635 (-2.1136, 24.684) -> (-2.1372, 24.6469)
  line L636 (-2.1372, 24.6469) -> (-2.1602, 24.6094)
  line L637 (-2.1602, 24.6094) -> (-2.1825, 24.5715)
  line L638 (-2.1825, 24.5715) -> (-2.2042, 24.5333)
  line L639 (-2.2042, 24.5333) -> (-2.2252, 24.4946)
  line L640 (-2.2252, 24.4946) -> (-2.2455, 24.4556)
  line L641 (-2.2455, 24.4556) -> (-2.2651, 24.4162)
  line L642 (-2.2651, 24.4162) -> (-2.284, 24.3765)
  line L643 (-2.284, 24.3765) -> (-2.3023, 24.3365)
  line L644 (-2.3023, 24.3365) -> (-2.3198, 24.2962)
  line L645 (-2.3198, 24.2962) -> (-2.3366, 24.2555)
  line L646 (-2.3366, 24.2555) -> (-2.3528, 24.2146)
  line L647 (-2.3528, 24.2146) -> (-2.3682, 24.1734)
  line L648 (-2.3682, 24.1734) -> (-2.3829, 24.1319)
  line L649 (-2.3829, 24.1319) -> (-2.3968, 24.0902)
  line L650 (-2.3968, 24.0902) -> (-2.41, 24.0483)
  line L651 (-2.41, 24.0483) -> (-2.4225, 24.0061)
  line L652 (-2.4225, 24.0061) -> (-2.4343, 23.9637)
  line L653 (-2.4343, 23.9637) -> (-2.4453, 23.9211)
  line L654 (-2.4453, 23.9211) -> (-2.4556, 23.8784)
  line L655 (-2.4556, 23.8784) -> (-2.4651, 23.8354)
  line L656 (-2.4651, 23.8354) -> (-2.4739, 23.7923)
  line L657 (-2.4739, 23.7923) -> (-2.4819, 23.7491)
  line L658 (-2.4819, 23.7491) -> (-2.4891, 23.7057)
  line L659 (-2.4891, 23.7057) -> (-2.4956, 23.6622)
  line L660 (-2.4956, 23.6622) -> (-2.5014, 23.6186)
  line L661 (-2.5014, 23.6186) -> (-2.5063, 23.5749)
  line L662 (-2.5063, 23.5749) -> (-2.5106, 23.5311)
  line L663 (-2.5106, 23.5311) -> (-2.514, 23.4872)
  line L664 (-2.514, 23.4872) -> (-2.5167, 23.4433)
  line L665 (-2.5167, 23.4433) -> (-2.5186, 23.3994)
  line L666 (-2.5186, 23.3994) -> (-2.5198, 23.3554)
  line L667 (-2.5198, 23.3554) -> (-2.5202, 23.3114)
  line L668 (-2.5202, 23.3114) -> (-2.5198, 23.2675)
  line L669 (-2.5198, 23.2675) -> (-2.5186, 23.2235)
  line L670 (-2.5186, 23.2235) -> (-2.5167, 23.1795)
  line L671 (-2.5167, 23.1795) -> (-2.514, 23.1356)
  line L672 (-2.514, 23.1356) -> (-2.5106, 23.0918)
  line L673 (-2.5106, 23.0918) -> (-2.5063, 23.048)
  line L674 (-2.5063, 23.048) -> (-2.5014, 23.0043)
  line L675 (-2.5014, 23.0043) -> (-2.4956, 22.9607)
  line L676 (-2.4956, 22.9607) -> (-2.4891, 22.9172)
  line L677 (-2.4891, 22.9172) -> (-2.4819, 22.8738)
  line L678 (-2.4819, 22.8738) -> (-2.4739, 22.8306)
  line L679 (-2.4739, 22.8306) -> (-2.4651, 22.7875)
  line L680 (-2.4651, 22.7875) -> (-2.4556, 22.7445)
  line L681 (-2.4556, 22.7445) -> (-2.4453, 22.7018)
  line L682 (-2.4453, 22.7018) -> (-2.4343, 22.6592)
  line L683 (-2.4343, 22.6592) -> (-2.4225, 22.6168)
  line L684 (-2.4225, 22.6168) -> (-2.41, 22.5746)
  line L685 (-2.41, 22.5746) -> (-2.3968, 22.5327)
  line L686 (-2.3968, 22.5327) -> (-2.3829, 22.491)
  line L687 (-2.3829, 22.491) -> (-2.3682, 22.4495)
  line L688 (-2.3682, 22.4495) -> (-2.3528, 22.4083)
  line L689 (-2.3528, 22.4083) -> (-2.3366, 22.3674)
  line L690 (-2.3366, 22.3674) -> (-2.3198, 22.3267)
  line L691 (-2.3198, 22.3267) -> (-2.3023, 22.2864)
  line L692 (-2.3023, 22.2864) -> (-2.284, 22.2464)
  line L693 (-2.284, 22.2464) -> (-2.2651, 22.2067)
  line L694 (-2.2651, 22.2067) -> (-2.2455, 22.1673)
  line L695 (-2.2455, 22.1673) -> (-2.2252, 22.1283)
  line L696 (-2.2252, 22.1283) -> (-2.2042, 22.0896)
  line L697 (-2.2042, 22.0896) -> (-2.1825, 22.0514)
  line L698 (-2.1825, 22.0514) -> (-2.1602, 22.0135)
  line L699 (-2.1602, 22.0135) -> (-2.1372, 21.976)
  line L700 (-2.1372, 21.976) -> (-0.315, 19.1018)
  line L701 (-0.315, 19.1018) -> (-0.315, 4.2097)
  line L702 (-0.315, 4.2097) -> (-2.1372, 1.3355)
  line L703 (-2.1372, 1.3355) -> (-2.1602, 1.298)
  line L704 (-2.1602, 1.298) -> (-2.1825, 1.2601)
  line L705 (-2.1825, 1.2601) -> (-2.2042, 1.2218)
  line L706 (-2.2042, 1.2218) -> (-2.2252, 1.1831)
  line L707 (-2.2252, 1.1831) -> (-2.2455, 1.1441)
  line L708 (-2.2455, 1.1441) -> (-2.2651, 1.1048)
  line L709 (-2.2651, 1.1048) -> (-2.284, 1.0651)
  line L710 (-2.284, 1.0651) -> (-2.3023, 1.025)
  line L711 (-2.3023, 1.025) -> (-2.3198, 0.9847)
  line L712 (-2.3198, 0.9847) -> (-2.3366, 0.9441)
  line L713 (-2.3366, 0.9441) -> (-2.3528, 0.9031)
  line L714 (-2.3528, 0.9031) -> (-2.3682, 0.8619)
  line L715 (-2.3682, 0.8619) -> (-2.3829, 0.8205)
  line L716 (-2.3829, 0.8205) -> (-2.3968, 0.7788)
  line L717 (-2.3968, 0.7788) -> (-2.41, 0.7368)
  line L718 (-2.41, 0.7368) -> (-2.4225, 0.6946)
  line L719 (-2.4225, 0.6946) -> (-2.4343, 0.6523)
  line L720 (-2.4343, 0.6523) -> (-2.4453, 0.6097)
  line L721 (-2.4453, 0.6097) -> (-2.4556, 0.5669)
  line L722 (-2.4556, 0.5669) -> (-2.4651, 0.524)
  line L723 (-2.4651, 0.524) -> (-2.4739, 0.4809)
  line L724 (-2.4739, 0.4809) -> (-2.4819, 0.4376)
  line L725 (-2.4819, 0.4376) -> (-2.4891, 0.3942)
  line L726 (-2.4891, 0.3942) -> (-2.4956, 0.3507)
  line L727 (-2.4956, 0.3507) -> (-2.5014, 0.3071)
  line L728 (-2.5014, 0.3071) -> (-2.5063, 0.2634)
  line L729 (-2.5063, 0.2634) -> (-2.5106, 0.2196)
  line L730 (-2.5106, 0.2196) -> (-2.514, 0.1758)
  line L731 (-2.514, 0.1758) -> (-2.5167, 0.1319)
  line L732 (-2.5167, 0.1319) -> (-2.5186, 0.088)
  line L733 (-2.5186, 0.088) -> (-2.5198, 0.044)
  line L734 (-2.5198, 0.044) -> (-2.5202, 0)
  line L735 (-2.5202, 0) -> (-2.5198, -0.044)
  line L736 (-2.5198, -0.044) -> (-2.5186, -0.088)
  line L737 (-2.5186, -0.088) -> (-2.5167, -0.1319)
  line L738 (-2.5167, -0.1319) -> (-2.514, -0.1758)
  line L739 (-2.514, -0.1758) -> (-2.5106, -0.2196)
  line L740 (-2.5106, -0.2196) -> (-2.5063, -0.2634)
  line L741 (-2.5063, -0.2634) -> (-2.5014, -0.3071)
  line L742 (-2.5014, -0.3071) -> (-2.4956, -0.3507)
  line L743 (-2.4956, -0.3507) -> (-2.4891, -0.3942)
  line L744 (-2.4891, -0.3942) -> (-2.4819, -0.4376)
  line L745 (-2.4819, -0.4376) -> (-2.4739, -0.4809)
  line L746 (-2.4739, -0.4809) -> (-2.4651, -0.524)
  line L747 (-2.4651, -0.524) -> (-2.4556, -0.5669)
  line L748 (-2.4556, -0.5669) -> (-2.4453, -0.6097)
  line L749 (-2.4453, -0.6097) -> (-2.4343, -0.6523)
  line L750 (-2.4343, -0.6523) -> (-2.4225, -0.6946)
  line L751 (-2.4225, -0.6946) -> (-2.41, -0.7368)
  line L752 (-2.41, -0.7368) -> (-2.3968, -0.7788)
  line L753 (-2.3968, -0.7788) -> (-2.3829, -0.8205)
  line L754 (-2.3829, -0.8205) -> (-2.3682, -0.8619)
  line L755 (-2.3682, -0.8619) -> (-2.3528, -0.9031)
  line L756 (-2.3528, -0.9031) -> (-2.3366, -0.9441)
  line L757 (-2.3366, -0.9441) -> (-2.3198, -0.9847)
  line L758 (-2.3198, -0.9847) -> (-2.3023, -1.025)
  line L759 (-2.3023, -1.025) -> (-2.284, -1.0651)
  line L760 (-2.284, -1.0651) -> (-2.2651, -1.1048)
  line L761 (-2.2651, -1.1048) -> (-2.2455, -1.1441)
  line L762 (-2.2455, -1.1441) -> (-2.2252, -1.1831)
  line L763 (-2.2252, -1.1831) -> (-2.2042, -1.2218)
  line L764 (-2.2042, -1.2218) -> (-2.1825, -1.2601)
  line L765 (-2.1825, -1.2601) -> (-2.1602, -1.298)
  line L766 (-2.1602, -1.298) -> (-2.1372, -1.3355)
  line L767 (-2.1372, -1.3355) -> (-2.1136, -1.3726)
  line L768 (-2.1136, -1.3726) -> (-2.0893, -1.4093)
  line L769 (-2.0893, -1.4093) -> (-2.0644, -1.4455)
  line L770 (-2.0644, -1.4455) -> (-2.0389, -1.4813)
  line L771 (-2.0389, -1.4813) -> (-2.0127, -1.5167)
  line L772 (-2.0127, -1.5167) -> (-1.9859, -1.5516)
  line L773 (-1.9859, -1.5516) -> (-1.9585, -1.586)
  line L774 (-1.9585, -1.586) -> (-1.9306, -1.6199)
  line L775 (-1.9306, -1.6199) -> (-1.902, -1.6534)
  line L776 (-1.902, -1.6534) -> (-1.8728, -1.6863)
  line L777 (-1.8728, -1.6863) -> (-1.8431, -1.7187)
  line L778 (-1.8431, -1.7187) -> (-1.8128, -1.7506)
  line L779 (-1.8128, -1.7506) -> (-1.782, -1.782)
  line L780 (-1.782, -1.782) -> (-1.7506, -1.8128)
  line L781 (-1.7506, -1.8128) -> (-1.7187, -1.8431)
  line L782 (-1.7187, -1.8431) -> (-1.6863, -1.8728)
  line L783 (-1.6863, -1.8728) -> (-1.6534, -1.902)
  line L784 (-1.6534, -1.902) -> (-1.6199, -1.9306)
  line L785 (-1.6199, -1.9306) -> (-1.586, -1.9585)
  line L786 (-1.586, -1.9585) -> (-1.5516, -1.9859)
  line L787 (-1.5516, -1.9859) -> (-1.5167, -2.0127)
  line L788 (-1.5167, -2.0127) -> (-1.4813, -2.0389)
  line L789 (-1.4813, -2.0389) -> (-1.4455, -2.0644)
  line L790 (-1.4455, -2.0644) -> (-1.4093, -2.0893)
  line L791 (-1.4093, -2.0893) -> (-1.3726, -2.1136)
  line L792 (-1.3726, -2.1136) -> (-1.3355, -2.1372)
  line L793 (-1.3355, -2.1372) -> (-1.298, -2.1602)
  line L794 (-1.298, -2.1602) -> (-1.2601, -2.1825)
  line L795 (-1.2601, -2.1825) -> (-1.2218, -2.2042)
  line L796 (-1.2218, -2.2042) -> (-1.1831, -2.2252)
  line L797 (-1.1831, -2.2252) -> (-1.1441, -2.2455)
  line L798 (-1.1441, -2.2455) -> (-1.1048, -2.2651)
  line L799 (-1.1048, -2.2651) -> (-1.0651, -2.284)
  line L800 (-1.0651, -2.284) -> (-1.025, -2.3023)
  line L801 (-1.025, -2.3023) -> (-0.9847, -2.3198)
  line L802 (-0.9847, -2.3198) -> (-0.9441, -2.3366)
  line L803 (-0.9441, -2.3366) -> (-0.9031, -2.3528)
  line L804 (-0.9031, -2.3528) -> (-0.8619, -2.3682)
  line L805 (-0.8619, -2.3682) -> (-0.8205, -2.3829)
  line L806 (-0.8205, -2.3829) -> (-0.7788, -2.3968)
  line L807 (-0.7788, -2.3968) -> (-0.7368, -2.41)
  line L808 (-0.7368, -2.41) -> (-0.6946, -2.4225)
  line L809 (-0.6946, -2.4225) -> (-0.6523, -2.4343)
  line L810 (-0.6523, -2.4343) -> (-0.6097, -2.4453)
  line L811 (-0.6097, -2.4453) -> (-0.5669, -2.4556)
  line L812 (-0.5669, -2.4556) -> (-0.524, -2.4651)
  line L813 (-0.524, -2.4651) -> (-0.4809, -2.4739)
  line L814 (-0.4809, -2.4739) -> (-0.4376, -2.4819)
  line L815 (-0.4376, -2.4819) -> (-0.3942, -2.4891)
  line L816 (-0.3942, -2.4891) -> (-0.3507, -2.4956)
  line L817 (-0.3507, -2.4956) -> (-0.3071, -2.5014)
  line L818 (-0.3071, -2.5014) -> (-0.2634, -2.5063)
  line L819 (-0.2634, -2.5063) -> (-0.2196, -2.5106)
  line L820 (-0.2196, -2.5106) -> (-0.1758, -2.514)
  line L821 (-0.1758, -2.514) -> (-0.1319, -2.5167)
  line L822 (-0.1319, -2.5167) -> (-0.088, -2.5186)
  line L823 (-0.088, -2.5186) -> (-0.044, -2.5198)
  line L824 (-0.044, -2.5198) -> (0, -2.5202)
  line L825 (0, -2.5202) -> (0.044, -2.5198)
  line L826 (0.044, -2.5198) -> (0.088, -2.5186)
  line L827 (0.088, -2.5186) -> (0.1319, -2.5167)
  line L828 (0.1319, -2.5167) -> (0.1758, -2.514)
  line L829 (0.1758, -2.514) -> (0.2196, -2.5106)
  line L830 (0.2196, -2.5106) -> (0.2634, -2.5063)
  line L831 (0.2634, -2.5063) -> (0.3071, -2.5014)
  line L832 (0.3071, -2.5014) -> (0.3507, -2.4956)
  line L833 (0.3507, -2.4956) -> (0.3942, -2.4891)
  line L834 (0.3942, -2.4891) -> (0.4376, -2.4819)
  line L835 (0.4376, -2.4819) -> (0.4809, -2.4739)
  line L836 (0.4809, -2.4739) -> (0.524, -2.4651)
  line L837 (0.524, -2.4651) -> (0.5669, -2.4556)
  line L838 (0.5669, -2.4556) -> (0.6097, -2.4453)
  line L839 (0.6097, -2.4453) -> (0.6523, -2.4343)
  line L840 (0.6523, -2.4343) -> (0.6946, -2.4225)
  line L841 (0.6946, -2.4225) -> (0.7368, -2.41)
  line L842 (0.7368, -2.41) -> (0.7788, -2.3968)
  line L843 (0.7788, -2.3968) -> (0.8205, -2.3829)
  line L844 (0.8205, -2.3829) -> (0.8619, -2.3682)
  line L845 (0.8619, -2.3682) -> (0.9031, -2.3528)
  line L846 (0.9031, -2.3528) -> (0.9441, -2.3366)
  line L847 (0.9441, -2.3366) -> (0.9847, -2.3198)
  line L848 (0.9847, -2.3198) -> (1.025, -2.3023)
  line L849 (1.025, -2.3023) -> (1.0651, -2.284)
  line L850 (1.0651, -2.284) -> (1.1048, -2.2651)
  line L851 (1.1048, -2.2651) -> (1.1441, -2.2455)
  line L852 (1.1441, -2.2455) -> (1.1831, -2.2252)
  line L853 (1.1831, -2.2252) -> (1.2218, -2.2042)
  line L854 (1.2218, -2.2042) -> (1.2601, -2.1825)
  line L855 (1.2601, -2.1825) -> (1.298, -2.1602)
  line L856 (1.298, -2.1602) -> (1.3355, -2.1372)
  line L857 (1.3355, -2.1372) -> (1.3726, -2.1136)
  line L858 (1.3726, -2.1136) -> (1.4093, -2.0893)
  line L859 (1.4093, -2.0893) -> (1.4455, -2.0644)
  line L860 (1.4455, -2.0644) -> (1.4813, -2.0389)
  line L861 (1.4813, -2.0389) -> (1.5167, -2.0127)
  line L862 (1.5167, -2.0127) -> (1.5516, -1.9859)
  line L863 (1.5516, -1.9859) -> (1.586, -1.9585)
  line L864 (1.586, -1.9585) -> (1.6199, -1.9306)
  line L865 (1.6199, -1.9306) -> (1.6534, -1.902)
  line L866 (1.6534, -1.902) -> (1.6863, -1.8728)
  line L867 (1.6863, -1.8728) -> (1.7187, -1.8431)
  line L868 (1.7187, -1.8431) -> (1.7506, -1.8128)
  line L869 (1.7506, -1.8128) -> (7.2526, 3.5702)
  line L870 (7.2526, 3.5702) -> (10.5007, 3.5702)
  line L871 (10.5007, 3.5702) -> (31.292, -17.2211)
  line L872 (31.292, -17.2211) -> (31.292, -23.1014)
  line L873 (31.292, -23.1014) -> (31.292, -23.1161)
  line L874 (31.292, -23.1161) -> (31.2925, -23.1307)
  line L875 (31.2925, -23.1307) -> (31.2931, -23.1454)
  line L876 (31.2931, -23.1454) -> (31.2939, -23.16)
  line L877 (31.2939, -23.16) -> (31.2952, -23.1746)
  line L878 (31.2952, -23.1746) -> (31.2965, -23.1892)
  line L879 (31.2965, -23.1892) -> (31.2981, -23.2038)
  line L880 (31.2981, -23.2038) -> (31.3002, -23.2184)
  line L881 (31.3002, -23.2184) -> (31.3023, -23.2328)
  line L882 (31.3023, -23.2328) -> (31.3047, -23.2473)
  line L883 (31.3047, -23.2473) -> (31.3074, -23.2617)
  line L884 (31.3074, -23.2617) -> (31.3103, -23.2761)
  line L885 (31.3103, -23.2761) -> (31.3134, -23.2904)
  line L886 (31.3134, -23.2904) -> (31.3169, -23.3047)
  line L887 (31.3169, -23.3047) -> (31.3206, -23.3188)
  line L888 (31.3206, -23.3188) -> (31.3245, -23.333)
  line L889 (31.3245, -23.333) -> (31.3285, -23.347)
  line L890 (31.3285, -23.347) -> (31.333, -23.361)
  line L891 (31.333, -23.361) -> (31.3378, -23.3749)
  line L892 (31.3378, -23.3749) -> (31.3425, -23.3887)
  line L893 (31.3425, -23.3887) -> (31.3478, -23.4025)
  line L894 (31.3478, -23.4025) -> (31.3531, -23.4161)
  line L895 (31.3531, -23.4161) -> (31.3587, -23.4297)
  line L896 (31.3587, -23.4297) -> (31.3645, -23.4431)
  line L897 (31.3645, -23.4431) -> (31.3706, -23.4564)
  line L898 (31.3706, -23.4564) -> (31.3769, -23.4697)
  line L899 (31.3769, -23.4697) -> (31.3836, -23.4828)
  line L900 (31.3836, -23.4828) -> (31.3902, -23.4958)
  line L901 (31.3902, -23.4958) -> (31.3973, -23.5087)
  line L902 (31.3973, -23.5087) -> (31.4045, -23.5215)
  line L903 (31.4045, -23.5215) -> (31.4119, -23.5341)
  line L904 (31.4119, -23.5341) -> (31.4195, -23.5466)
  line L905 (31.4195, -23.5466) -> (31.4275, -23.559)
  line L906 (31.4275, -23.559) -> (31.4357, -23.5712)
  line L907 (31.4357, -23.5712) -> (31.4439, -23.5833)
  line L908 (31.4439, -23.5833) -> (31.4523, -23.5952)
  line L909 (31.4523, -23.5952) -> (31.4611, -23.607)
  line L910 (31.4611, -23.607) -> (31.4701, -23.6186)
  line L911 (31.4701, -23.6186) -> (31.4791, -23.6301)
  line L912 (31.4791, -23.6301) -> (31.4886, -23.6414)
  line L913 (31.4886, -23.6414) -> (31.4981, -23.6526)
  line L914 (31.4981, -23.6526) -> (31.5076, -23.6635)
  line L915 (31.5076, -23.6635) -> (31.5177, -23.6743)
  line L916 (31.5177, -23.6743) -> (31.5278, -23.685)
  line L917 (31.5278, -23.685) -> (31.5381, -23.6954)
  line L918 (31.5381, -23.6954) -> (31.5484, -23.7057)
  line L919 (31.5484, -23.7057) -> (31.559, -23.7158)
  line L920 (31.559, -23.7158) -> (31.5698, -23.7257)
  line L921 (31.5698, -23.7257) -> (31.5809, -23.7354)
  line L922 (31.5809, -23.7354) -> (31.592, -23.745)
  line L923 (31.592, -23.745) -> (31.6034, -23.7543)
  line L924 (31.6034, -23.7543) -> (31.6148, -23.7634)
  line L925 (31.6148, -23.7634) -> (31.6264, -23.7723)
  line L926 (31.6264, -23.7723) -> (31.6383, -23.781)
  line L927 (31.6383, -23.781) -> (31.6503, -23.7896)
  line L928 (31.6503, -23.7896) -> (31.6622, -23.7979)
  line L929 (31.6622, -23.7979) -> (31.6746, -23.806)
  line L930 (31.6746, -23.806) -> (31.6868, -23.8138)
  line L931 (31.6868, -23.8138) -> (31.6995, -23.8215)
  line L932 (31.6995, -23.8215) -> (31.7119, -23.8289)
  line L933 (31.7119, -23.8289) -> (31.7246, -23.8362)
  line L934 (31.7246, -23.8362) -> (31.7376, -23.8431)
  line L935 (31.7376, -23.8431) -> (31.7505, -23.8499)
  line L936 (31.7505, -23.8499) -> (31.7638, -23.8565)
  line L937 (31.7638, -23.8565) -> (31.777, -23.8628)
  line L938 (31.777, -23.8628) -> (31.7902, -23.8689)
  line L939 (31.7902, -23.8689) -> (31.8037, -23.8747)
  line L940 (31.8037, -23.8747) -> (31.8172, -23.8803)
  line L941 (31.8172, -23.8803) -> (31.831, -23.8857)
  line L942 (31.831, -23.8857) -> (31.8447, -23.8908)
  line L943 (31.8447, -23.8908) -> (31.8585, -23.8957)
  line L944 (31.8585, -23.8957) -> (31.8725, -23.9004)